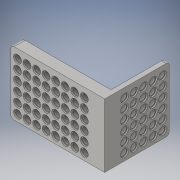
# Autodesk Inventor part: angle_plate
Saved by Autodesk Inventor 2016 (Build 200138000, 138)
## iProperties
Created: 2016-02-13
Part Number: angle_plate
Material: Generic
Document SubType Name: Modeling
Designer: jforce
Density: 1 g/cm^3
Appearance: Default
Author: jforce
Autodesk Inventor part; units mm, degrees
ref_plane "YZ Plane" through (0, 0, 0) normal (1, 0, 0) x (0, 1, 0)
ref_plane "XZ Plane" through (0, 0, 0) normal (0, 1, 0) x (-1, 0, 0)
ref_plane "XY Plane" through (0, 0, 0) normal (0, 0, 1) x (1, 0, 0)
sketch "Sketch1" plane through (0, 0, 0) normal (0, 0, 1) x (1, 0, 0)
  line L0 (2, 0) -> (56, 0)
  line L1 (56, 0) -> (56, 40)
  line L2 (56, 40) -> (2, 40)
  line L3 (0, 38) -> (0, 2)
  arc A0 (2, 40) -> (0, 38) centre (2, 38) ccw
  arc A1 (0, 2) -> (2, 0) centre (2, 2) ccw
  point P0 (0, 0)
  point P1 (0, 40)
  dimension "d0" = 56
  dimension "d1" = 40
  constraints: 8 end point, 4 point on circle, 4 point on line, 4 tangent, 2 centre point, 2 parallel, 1 horizontal, 1 perpendicular
  measures "d0" distance of L1.end point (0, 40)
  measures "d1" distance of L0.end L1.end
extrude "Extrusion1" add sketch "Sketch1" along normal blind 7
sketch "Sketch2" plane through (0, 0, 7) normal (0, 0, 1) x (1, 0, 0)
  point P0 (0, 0)
  point P1 (4.2467, 4.3978)
hole "Hole1" at (4.2467, 4.3978, 7) direction (0, 0, -1) diameter 4 depth 7 tip angle 118 counterbore diameter 5 counterbore depth 0.85
sketch "Sketch3" plane through (0, 0, 0) normal (0, 0, -1) x (-1, 0, 0)
  circle A0 centre (-4.2467, 4.3978) radius 2 projected
  circle A1 centre (-4.2467, 4.3978) radius 2.5
  point P0 (0, 0)
  dimension "d12" = 5
  constraints: 1 centre point, 1 coincident
  measures "d12" diameter of A1
extrude "Extrusion2" cut sketch "Sketch3" against normal blind 0.85
pattern_linear "Rectangular Pattern1" count 8 spacing 6 along (1, 0, 0) count 6 spacing 6 along (0, 1, 0) of "Hole1", "Extrusion2"
sketch "Sketch4" plane through (56, 0, 0) normal (1, 0, 0) x (0, 0, -1)
  line L0 (0, 0) -> (0, 40) projected
  line L1 (0, 40) -> (-7, 40) projected
  line L2 (-7, 0) -> (-7, 40) projected
  line L3 (0, 0) -> (-7, 0) projected
  line L4 (-7, 40) -> (31.5867, 40)
  line L5 (33.5867, 38) -> (33.5867, 2)
  line L6 (31.5867, 0) -> (-7, 0)
  arc A0 (33.5867, 38) -> (31.5867, 40) centre (31.5867, 38) ccw
  arc A1 (31.5867, 0) -> (33.5867, 2) centre (31.5867, 2) ccw
  line L7 (-7, 0) -> (-7, 40) projected
  line L8 (-7, 40) -> (-7, 0)
  point P0 (0, 0)
  point P1 (33.5867, 0)
  point P2 (33.5867, 40)
  dimension "d37" = 2
  constraints: 8 end point, 6 point on line, 4 point on circle, 4 tangent, 2 centre point, 2 equal length, 1 equal radius, 1 horizontal, 1 perpendicular
  measures "d37" radius of A0
extrude "Extrusion3" add sketch "Sketch4" along normal blind 3
sketch "Sketch6" plane through (59, 0, 0) normal (1, 0, 0) x (0, 0, -1)
  line L0 (0, 40) -> (-7, 40) projected
  line L1 (-3.5, 40) -> (-3.5, 0) construction
  line L2 (-7, 0) -> (31.5867, 0) projected
  line L3 (-0.85, 6.3978) -> (-0.85, 2.3978) projected
  line L4 (-6.15, 6.3978) -> (-6.15, 2.3978) projected
  line L5 (-3.5, 4.3978) -> (5.5, 4.3978) construction
  point P0 (0, 0)
  dimension "d44" = 9
  constraints: 4 end point, 2 point on line, 1 midpoint, 1 vertical
  measures "d44" distance of L5.start L5.end
hole "Hole3" at (59, 4.3978, -5.5) direction (-1, 0, 0) diameter 4 depth 3 tip angle 118 counterbore diameter 5 counterbore depth 0.85
pattern_linear "Rectangular Pattern4" count 6 spacing 6 along (0, 1, 0) count 5 spacing 6 along (0, 0, -1) of "Hole3"
body "Solid1"
